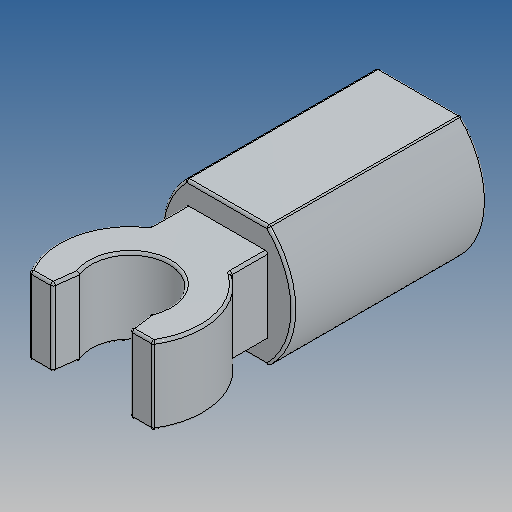
# Autodesk Inventor part: 44873-LtBluishGray
Saved by Autodesk Inventor 2025 (Build 290162010, 162A)
## iProperties
Created: 2014-09-17
Part Number: 44873-LtBluishGray
Material: ABS Plastic
Document SubType Name: Modeling
Designer: D. Kohfeld
Mass: 0.232563 g
Surface Area: 3.25413 cm^2
Volume: 0.219399 cm^3
Density: 1.06 g/cm^3
Appearance: LtBluishGray
Author: D. Kohfeld
Autodesk Inventor part; units mm, degrees
ref_plane "YZ Plane" through (0, 0, 0) normal (1, 0, 0) x (0, 1, 0)
ref_plane "XZ Plane" through (0, 0, 0) normal (0, 1, 0) x (-1, 0, 0)
ref_plane "XY Plane" through (0, 0, 0) normal (0, 0, 1) x (1, 0, 0)
sketch "Sketch2" plane through (0, 0, 0) normal (0, 0, 1) x (1, 0, 0)
  line L0 (-1.695, 2.5) -> (1.695, 2.5)
  line L1 (-1.695, -2.5) -> (1.695, -2.5)
  arc A0 (1.695, -2.5) -> (1.695, 2.5) centre (-0.7562, 0) ccw
  arc A1 (-1.695, 2.5) -> (-1.695, -2.5) centre (0.7562, 0) ccw
  circle A2 centre (0, 0) radius 1.6
  line L2 (-0.7562, 0) -> (0.7562, 0) construction
  dimension "d0" = 5
  dimension "d2" = 3.2
  dimension "d7" = 3.39
  dimension "d9" = 5.49
  constraints: 6 end point, 4 point on circle, 3 centre point, 3 parallel, 2 coincident, 2 horizontal alignment, 1 equal radius, 1 horizontal, 1 midpoint
  measures "d0" distance between parallel lines of L0 L1
  measures "d2" diameter of A2
  measures "d7" distance of L0.start L0.end
extrude "Extrusion1" add sketch "Sketch2" along normal blind 8 contours L0 A0 L1 A1 | A2
extrude "Extrusion2" cut sketch "Sketch2" along normal blind 4 contours A2
sketch "Sketch3" plane through (0, 0, 0) normal (0, 1, 0) x (-1, 0, 0)
  line L0 (-1.695, 8) -> (1.695, 8) construction
  line L1 (-1.6765, 8) -> (1.6765, 8)
  line L2 (1.6765, 8) -> (1.6765, 9.5122)
  line L3 (-1.6765, 8) -> (-1.6765, 9.5122)
  arc A0 (-2.5377, 13.6) -> (-1.6765, 9.5122) centre (0, 12) ccw
  arc A1 (1.6765, 9.5122) -> (2.5377, 13.6) centre (0, 12) ccw
  line L4 (-2.5377, 13.6) -> (-1.6, 13.6)
  line L5 (-1.6, 13.6) -> (-1.475, 12.62)
  line L6 (2.5377, 13.6) -> (1.6, 13.6)
  line L7 (1.6, 13.6) -> (1.475, 12.62)
  arc A2 (-1.475, 12.62) -> (1.475, 12.62) centre (0, 12) ccw
  point P0 (0, 0)
  point P1 (0, 8)
  dimension "d10" = 3.2
  dimension "d11" = 2.95
  dimension "d12" = 3.2
  dimension "d13" = 5.6
  dimension "d14" = 4
  dimension "d16" = 3.353
  dimension "d17" = 6
  constraints: 14 end point, 6 point on circle, 3 centre point, 3 equal length, 2 coincident, 2 midpoint, 2 perpendicular, 1 horizontal, 1 horizontal alignment, 1 parallel, 1 point on line, 1 vertical alignment
  measures "d10" diameter of A2
  measures "d11" distance of L7.end L5.end
  measures "d12" distance of L6.end L4.end
  measures "d13" distance between parallel lines of L4 L1
  measures "d14" distance from line of L1 A2.centre
  measures "d16" distance between parallel lines of L2 L3
  measures "d17" diameter of A0
extrude "Extrusion3" add sketch "Sketch3" along normal mid plane 3.2
fillet "Fillet1" radius 0.1 36 edges at (-1.5375, 1.6, 13.11) (-2.0689, 1.6, 13.6) (-2.5377, 0, 13.6) (-1.6, 0, 13.6) (-2.0689, -1.6, 13.6) (-2.9356, 1.6, 11.3815) (-2.9356, -1.6, 11.3815) (0, 1.6, 10.4) (0, -1.6, 10.4) (-1.5375, -1.6, 13.11) (1.5375, -1.6, 13.11) (1.6, 0, 13.6) (1.5375, 1.6, 13.11) (2.0689, 1.6, 13.6) (2.5377, 0, 13.6) (2.9356, 1.6, 11.3815) (2.0689, -1.6, 13.6) (2.9356, -1.6, 11.3815) (1.6765, 1.6, 8.7561) (-1.6765, 1.6, 8.7561) (-1.695, 2.5, 4) (1.6765, -1.6, 8.7561) (2.745, 0, 8) (0, 2.5, 8) (-2.745, 0, 8) (1.695, 2.5, 4) (0, -2.5, 8) (-1.6765, -1.6, 8.7561) (-1.695, -2.5, 4) (1.695, -2.5, 4) (0, -2.5, 0) (-2.745, 0, 0) (2.745, 0, 0) (0, 2.5, 0) (1.6765, 0, 9.5122) (-1.6765, 0, 9.5122)
equation "\"d2\" = rd"
equation "\"d3\" = lu"
equation "\"d5\" = 0.5 * lu"
equation "\"d10\" = rd"
equation "\"d12\" = rd"
equation "\"rd\" = 3.2"
equation "\"lu\" = 8"
body "Solid1"
